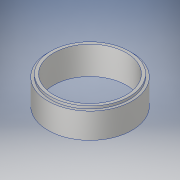
# Autodesk Inventor part: aluminum_retainer
Saved by Autodesk Inventor 2017 SP1 (Build 210196100, 196)
## iProperties
Created: 2016-10-22
Part Number: aluminum_retainer
Material: Aluminum 6061
Document SubType Name: Modeling
Designer: cflannery
Density: 2.7 g/cm^3
Appearance: Aluminum - Flat
Author: cflannery
Autodesk Inventor part; units mm, degrees
ref_plane "YZ Plane" through (0, 0, 0) normal (1, 0, 0) x (0, 1, 0)
ref_plane "XZ Plane" through (0, 0, 0) normal (0, 1, 0) x (-1, 0, 0)
ref_plane "XY Plane" through (0, 0, 0) normal (0, 0, 1) x (1, 0, 0)
sketch "Sketch1" plane through (0, 0, 0) normal (0, 0, 1) x (1, 0, 0)
  arc A0 (-28.9184, -1.6435) -> (-32.3684, 5.7551) centre (-35.052, 0) ccw
  line L0 (-28.702, 47.5942) -> (-28.702, -124.4009) construction
  line L1 (-32.3684, 5.7551) -> (-88.9, 32.1162)
  line L2 (-28.9184, -1.6435) -> (-86.2301, -215.5338)
  line L3 (-46.4564, 12.3244) -> (-66.802, 12.3244)
  line L4 (-60.4508, -95.6256) -> (-54.1008, -95.6256)
  line L5 (-73.152, -5.9838) -> (-73.152, -131.1779)
  line L6 (-73.152, -131.1779) -> (-63.627, -131.1779)
  line L7 (58.5667, 38.1) -> (-194.088, 38.1) construction
  line L8 (-95.25, 6.7162) -> (-95.25, -5.9838)
  line L9 (-95.25, 6.7162) -> (-88.9, 6.7162)
  line L10 (-88.9, 6.7162) -> (-88.9, 32.1162)
  line L11 (-95.25, -5.9838) -> (-73.152, -5.9838)
  line L12 (-95.25, -5.9838) -> (-95.25, -18.6838)
  line L13 (-95.25, -18.6838) -> (-89.3064, -18.6838)
  line L14 (-89.3064, -18.6838) -> (-89.3064, -24.6274)
  line L15 (-89.3064, -24.6274) -> (-95.25, -24.6274)
  line L16 (-95.25, -24.6274) -> (-95.25, -82.1838)
  line L17 (-95.25, -82.1838) -> (-82.55, -82.1838)
  line L18 (-89.3064, -18.6838) -> (-82.55, -18.6838)
  line L19 (-82.55, -18.6838) -> (-82.55, -82.1838)
  line L20 (-95.25, -82.1838) -> (-101.6, -82.1838)
  line L21 (-66.802, 12.3244) -> (-66.802, -31.3838)
  line L22 (-66.802, -31.3838) -> (-60.4508, -95.6256)
  line L23 (-82.55, -178.1009) -> (-76.2, -178.1009)
  line L24 (-82.55, -82.1838) -> (-82.55, -178.1009)
  line L25 (-86.2301, -215.5338) -> (-89.4051, -215.5338)
  line L26 (-89.4051, -215.5338) -> (-101.6, -82.1838)
  line L27 (-69.977, -5.9838) -> (-69.977, -31.3838)
  line L28 (-69.977, -31.3838) -> (-73.152, -31.3838)
  line L29 (-69.977, -5.9838) -> (-66.802, -5.9838)
  line L30 (-101.6, -82.1838) -> (-28.702, -82.1838) construction
  line L31 (0, -210.5351) -> (0, 86.485) construction
  point P0 (0, 0)
  dimension "d0" = 12.7
  dimension "d1" = 28.702
  dimension "d3" = 15
  dimension "d4" = 6.35
  dimension "d9" = 38.1
  dimension "d11" = 12.7
  dimension "d13" = 95.25
  dimension "d14" = 6.35
  dimension "d15" = 25.4
  dimension "d17" = 12.7
  dimension "d18" = 5.9436
  dimension "d19" = 5.9436
  dimension "d20" = 12.7
  dimension "d22" = 107.95
  dimension "d23" = 63.5
  dimension "d25" = 25.4
  dimension "d26" = 6.35
  dimension "d27" = 133.35
  dimension "d28" = 3.175
  dimension "d29" = 101.6
  dimension "d30" = 6.35
  dimension "d31" = 25
  dimension "d32" = 44.45
  dimension "d33" = 3.175
  dimension "d34" = 20.3456
  dimension "d35" = 9.525
  constraints: 64 end point, 11 perpendicular, 8 horizontal, 8 point on line, 7 vertical, 3 horizontal alignment, 3 point on circle, 3 tangent, 2 parallel, 1 centre point, 1 vertical alignment
  measures "d0" diameter of A0
  measures "d1" distance from line of point (0, 0) L0
  measures "d3" angle of L0 L2
  measures "d4" distance of L4.start L4.end
  measures "d9" distance from line of point (0, 0) L7
  measures "d11" distance of L8.start L8.end
  measures "d13" distance from line of point (0, 0) L8
  measures "d14" distance between parallel lines of L8 L10
  measures "d15" distance of L9.end L1.end
  measures "d17" distance of L8.end L12.end
  measures "d18" distance of L13.end L14.end
  measures "d19" distance of L12.end L13.end
  measures "d20" distance of L18.end L12.end
  measures "d22" distance between parallel lines of L4 L3
  measures "d23" distance between parallel lines of L13 L20
  measures "d25" distance from line of L21.end L11
  measures "d26" distance of L23.start L23.end
  measures "d27" distance between parallel lines of L20 L25
  measures "d28" distance of L2.end L25.end
  measures "d29" horizontal distance of point (0, 0) L20.end
  measures "d30" distance between parallel lines of L5 L21
  measures "d31" angle of L7 L1
  measures "d32" distance between parallel lines of L0 L5
  measures "d33" distance between parallel lines of L21 L27
  measures "d34" distance of L3.start L3.end
  measures "d35" distance of L5.end L6.end
revolve "Revolution2" add sketch "Sketch1" angle 360 about axis through (0, -210.5351, 0) along (0, 1, 0) contours L17 L16 L15 L14 L18 L19
body "Solid2"
